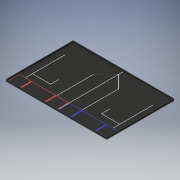
# Autodesk Inventor part: Field
Saved by Autodesk Inventor 2017 (Build 210142000, 142)
## iProperties
Created: 2017-04-14
Part Number: Field
Material: Generic
Document SubType Name: Modeling
Designer: Alex Tacescu
Density: 1 g/cm^3
Appearance: Rubber - Black
Author: Alex Tacescu
Autodesk Inventor part; units mm, degrees
ref_plane "YZ Plane" through (0, 0, 0) normal (1, 0, 0) x (0, 1, 0)
ref_plane "XZ Plane" through (0, 0, 0) normal (0, 1, 0) x (-1, 0, 0)
ref_plane "XY Plane" through (0, 0, 0) normal (0, 0, 1) x (1, 0, 0)
sketch "Sketch1" plane through (0, 0, 0) normal (0, 1, 0) x (-1, 0, 0)
  line L0 (0, -1706.88) -> (0, 1706.88) projected
  line L1 (-2560.32, 0) -> (2560.32, 0) projected
  line L2 (1828.8, 1219.2) -> (-1828.8, 1219.2)
  line L3 (-1828.8, 1219.2) -> (-1828.8, -1219.2)
  line L4 (-1828.8, -1219.2) -> (1828.8, -1219.2)
  line L5 (1828.8, -1219.2) -> (1828.8, 1219.2)
  line L6 (1828.8, 1219.2) -> (-1828.8, -1219.2) construction
  line L7 (-1828.8, 1219.2) -> (1828.8, -1219.2) construction
  point P0 (0, 0)
  dimension "d0" = 2438.4
  dimension "d1" = 3657.6
  constraints: 12 end point, 2 midpoint, 2 parallel, 1 horizontal, 1 perpendicular
  measures "d0" distance of L2.end L3.end
  measures "d1" distance of L3.end L4.end
extrude "Extrusion1" add sketch "Sketch1" along normal blind 6.35
sketch "Sketch2" plane through (0, 6.35, 0) normal (0, 1, 0) x (1, 0, 0)
  line L0 (-1828.8, -1219.2) -> (1828.8, -1219.2) projected
  line L1 (1828.8, -1219.2) -> (1828.8, 1219.2) projected
  line L2 (1828.8, 1219.2) -> (-1828.8, 1219.2) projected
  line L3 (-1828.8, 1219.2) -> (-1828.8, -1219.2) projected
  line L4 (-1816.1, 1206.5) -> (1816.1, 1206.5)
  line L5 (1816.1, 1206.5) -> (1816.1, -1206.5)
  line L6 (1816.1, -1206.5) -> (-1816.1, -1206.5)
  line L7 (-1816.1, -1206.5) -> (-1816.1, 1206.5)
  point P0 (0, 0)
  dimension "d4" = 12.7
  constraints: 8 end point, 3 other
  measures "d4" distance between parallel lines of L2 L4
extrude "Extrusion2" add sketch "Sketch2" along normal blind 63.5
sketch "Sketch4" plane through (0, 6.35, 0) normal (0, 1, 0) x (1, 0, 0)
  line L0 (1816.1, -1206.5) -> (1816.1, 1206.5) projected
  line L1 (1816.1, 1206.5) -> (-1816.1, 1206.5) projected
  line L2 (-1816.1, 1206.5) -> (-1816.1, -1206.5) projected
  line L3 (-1816.1, -1206.5) -> (1816.1, -1206.5) projected
  line L4 (-1828.8, -1219.2) -> (1828.8, -1219.2) projected
  line L5 (-1828.8, 1219.2) -> (-1828.8, -1219.2) projected
  line L6 (1828.8, 1219.2) -> (-1828.8, 1219.2) projected
  line L7 (1828.8, -1219.2) -> (1828.8, 1219.2) projected
  line L8 (-1816.1, -1206.5) -> (-1358.9, -1206.5)
  line L9 (-1358.9, -1206.5) -> (-1358.9, -749.3)
  line L10 (-1358.9, -749.3) -> (-1816.1, -749.3)
  line L11 (-1816.1, -749.3) -> (-1816.1, -1206.5)
  line L12 (-1790.7, -774.7) -> (-1384.3, -774.7)
  line L13 (-1384.3, -774.7) -> (-1384.3, -1181.1)
  line L14 (-1384.3, -1181.1) -> (-1790.7, -1181.1)
  line L15 (-1790.7, -1181.1) -> (-1790.7, -774.7)
  line L16 (0, 1706.88) -> (0, -1706.88) projected
  line L17 (2560.32, 0) -> (-2560.32, 0) projected
  line L18 (-1358.9, -1206.5) -> (-469.9, -1206.5)
  line L19 (-469.9, -1206.5) -> (-469.9, -749.3)
  line L20 (-469.9, -749.3) -> (-1358.9, -749.3)
  line L21 (-1358.9, -749.3) -> (-1358.9, -1206.5)
  line L22 (-469.9, -749.3) -> (-12.7, -749.3)
  line L23 (-12.7, -749.3) -> (-12.7, -1206.5)
  line L24 (-12.7, -1206.5) -> (-469.9, -1206.5)
  line L25 (-469.9, -1206.5) -> (-469.9, -749.3)
  line L26 (-495.3, -774.7) -> (-1333.5, -774.7)
  line L27 (-1333.5, -774.7) -> (-1333.5, -1181.1)
  line L28 (-1333.5, -1181.1) -> (-495.3, -1181.1)
  line L29 (-495.3, -1181.1) -> (-495.3, -774.7)
  line L30 (-444.5, -774.7) -> (-38.1, -774.7)
  line L31 (-38.1, -774.7) -> (-38.1, -1181.1)
  line L32 (-38.1, -1181.1) -> (-444.5, -1181.1)
  line L33 (-444.5, -1181.1) -> (-444.5, -774.7)
  line L34 (-12.7, -1206.5) -> (0, -1206.5)
  line L35 (0, -1206.5) -> (0, 609.6)
  line L36 (0, 609.6) -> (-12.7, 609.6)
  line L37 (-12.7, 609.6) -> (-12.7, -1206.5)
  line L38 (-1574.8, -749.3) -> (-1600.2, -749.3)
  point P0 (0, 0)
  dimension "d7" = 457.2
  dimension "d8" = 25.4
  dimension "d9" = 889
  dimension "d10" = 457.2
  dimension "d11" = 25.4
  dimension "d12" = 25.4
  dimension "d13" = 609.6
  constraints: 58 end point, 12 parallel, 8 perpendicular, 5 horizontal, 4 collinear, 3 point on line, 6 other
  measures "d7" distance of L8.end L9.end
  measures "d8" distance between parallel lines of L10 L12
  measures "d9" distance of L19.end L20.end
  measures "d10" distance of L19.end L22.end
  measures "d11" distance between parallel lines of L27 L9
  measures "d12" distance between parallel lines of L29 L25
  measures "d13" distance between parallel lines of L36 L6
extrude "Extrusion3" add sketch "Sketch4" along normal blind 0.254 contours L3 L19 L22 L23 | L3 L9 L20 L19 | L3 L2 L10 L9
sketch "Sketch7" plane through (0, 6.35, 0) normal (0, 1, 0) x (1, 0, 0)
  line L0 (0, 1706.88) -> (0, -1706.88) projected
  line L1 (2560.32, 0) -> (-2560.32, 0) projected
  line L2 (-1816.1, -749.3) -> (-12.7, -749.3) projected
  line L3 (-12.7, -749.3) -> (-12.7, -1206.5) projected
  line L4 (-12.7, -1206.5) -> (1816.1, -1206.5) projected
  line L5 (1816.1, -1206.5) -> (1816.1, 1206.5) projected
  line L6 (1816.1, 1206.5) -> (-1816.1, 1206.5) projected
  line L7 (-1816.1, 1206.5) -> (-1816.1, -749.3) projected
  line L8 (-469.9, 590.804) -> (-444.5, 590.804)
  line L9 (-444.5, 590.804) -> (-444.5, -749.046)
  line L10 (-444.5, -749.046) -> (-469.9, -749.046)
  line L11 (-469.9, -749.046) -> (-469.9, 590.804)
  line L12 (-469.9, 590.804) -> (-17.9605, 1042.7435)
  line L13 (-17.9605, 1042.7435) -> (0, 1024.783)
  line L14 (-444.5, -1181.1) -> (-444.5, -774.7) projected
  line L15 (0, 1024.783) -> (-444.5, 580.283)
  line L16 (-1600.2, -749.046) -> (-1574.8, -749.046)
  line L17 (-1574.8, -749.046) -> (-1574.8, 698.5)
  line L18 (-1574.8, 698.5) -> (-1600.2, 698.5)
  line L19 (-1600.2, 698.5) -> (-1600.2, -749.046)
  line L20 (-12.7, -749.3) -> (-1816.1, -749.3) projected
  line L21 (-1574.8, -520.7) -> (-914.4, -520.7)
  line L22 (-914.4, -520.7) -> (-914.4, -495.3)
  line L23 (-914.4, -495.3) -> (-1574.8, -495.3)
  line L24 (-1574.8, -495.3) -> (-1574.8, -520.7)
  line L25 (-914.4, -495.3) -> (-939.8, -495.3)
  line L26 (-939.8, -495.3) -> (-939.8, -209.55)
  line L27 (-939.8, -209.55) -> (-914.4, -209.55)
  line L28 (-914.4, -209.55) -> (-914.4, -495.3)
  point P0 (0, 0)
  dimension "d21" = 1339.85
  dimension "d22" = 25.4
  dimension "d23" = 0.254
  dimension "d24" = 135
  dimension "d25" = 508
  dimension "d26" = 0.254
  dimension "d27" = 215.9
  dimension "d28" = 228.6
  dimension "d29" = 285.75
  dimension "d31" = 635
  constraints: 38 end point, 9 parallel, 5 perpendicular, 4 equal length, 4 horizontal, 3 point on line, 1 collinear
  measures "d21" distance of L8.end L9.end
  measures "d22" distance of L9.end L10.end
  measures "d23" distance between parallel lines of L2 L10
  measures "d24" angle of L9 L15
  measures "d25" distance between parallel lines of L6 L18
  measures "d26" distance between parallel lines of L20 L16
  measures "d27" distance between parallel lines of L7 L19
  measures "d28" distance between parallel lines of L20 L21
  measures "d29" distance of L25.end L26.end
  measures "d31" distance between parallel lines of L17 L26
extrude "Extrusion5" add sketch "Sketch7" along normal blind 0.254 contours L15 L9 L8 L12 L13 | L9 L1 L11 L8 | L9 L10 L11 L1 | L19 L18 L17 L1 | L1 L17 L16 L19 | L23 L22 L21 L17 | L26 L27 L28 L23
mirror "Mirror1" about plane through (0, 0, 0) normal (1, 0, 0) of "Extrusion3", "Extrusion5"
sketch "Sketch5" plane through (0, 6.35, 0) normal (0, 1, 0) x (1, 0, 0)
  line L0 (-1384.3, -774.7) -> (-1384.3, -1181.1) projected
  line L1 (-1384.3, -1181.1) -> (-1790.7, -1181.1) projected
  line L2 (-1790.7, -1181.1) -> (-1790.7, -774.7) projected
  line L3 (-1790.7, -774.7) -> (-1384.3, -774.7) projected
  line L4 (-495.3, -774.7) -> (-495.3, -1181.1) projected
  line L5 (-495.3, -1181.1) -> (-1333.5, -1181.1) projected
  line L6 (-1333.5, -1181.1) -> (-1333.5, -774.7) projected
  line L7 (-1333.5, -774.7) -> (-495.3, -774.7) projected
  line L8 (-38.1, -774.7) -> (-38.1, -1181.1) projected
  line L9 (-38.1, -1181.1) -> (-444.5, -1181.1) projected
  line L10 (-444.5, -1181.1) -> (-444.5, -774.7) projected
  line L11 (-444.5, -774.7) -> (-38.1, -774.7) projected
  line L12 (-12.7, -1206.5) -> (-12.7, -749.3) projected
  line L13 (-12.7, -749.3) -> (-1816.1, -749.3) projected
  line L14 (-1816.1, -1206.5) -> (-1816.1, -749.3) projected
  line L15 (-12.7, -1206.5) -> (-1816.1, -1206.5) projected
  line L16 (1384.3, -774.7) -> (1384.3, -1181.1) projected
  line L17 (1790.7, -774.7) -> (1384.3, -774.7) projected
  line L18 (1790.7, -1181.1) -> (1790.7, -774.7) projected
  line L19 (1384.3, -1181.1) -> (1790.7, -1181.1) projected
  line L20 (495.3, -774.7) -> (495.3, -1181.1) projected
  line L21 (1333.5, -774.7) -> (495.3, -774.7) projected
  line L22 (1333.5, -1181.1) -> (1333.5, -774.7) projected
  line L23 (495.3, -1181.1) -> (1333.5, -1181.1) projected
  line L24 (38.1, -774.7) -> (38.1, -1181.1) projected
  line L25 (444.5, -774.7) -> (38.1, -774.7) projected
  line L26 (444.5, -1181.1) -> (444.5, -774.7) projected
  line L27 (38.1, -1181.1) -> (444.5, -1181.1) projected
  line L28 (12.7, -1206.5) -> (12.7, -749.3) projected
  line L29 (1816.1, -1206.5) -> (12.7, -1206.5) projected
  line L30 (1816.1, -749.3) -> (1816.1, -1206.5) projected
  line L31 (12.7, -749.3) -> (1816.1, -749.3) projected
  line L32 (12.7, -749.3) -> (1816.1, -749.3) projected
  line L33 (1816.1, -749.3) -> (1816.1, 1206.5) projected
  line L34 (1816.1, 1206.5) -> (-1816.1, 1206.5) projected
  line L35 (-1816.1, 1206.5) -> (-1816.1, -749.3) projected
  line L36 (-1816.1, -749.3) -> (-12.7, -749.3) projected
  line L37 (-12.7, -749.3) -> (-12.7, -1206.5) projected
  line L38 (-12.7, -1206.5) -> (12.7, -1206.5) projected
  line L39 (12.7, -1206.5) -> (12.7, -749.3) projected
  line L40 (-12.7, -1206.5) -> (12.7, -1206.5)
  line L41 (12.7, -1206.5) -> (12.7, 1206.5)
  line L42 (12.7, 1206.5) -> (-12.7, 1206.5)
  line L43 (-12.7, 1206.5) -> (-12.7, -1206.5)
  line L44 (-12.6746, -1206.4746) -> (12.6746, -1206.4746)
  line L45 (12.6746, -1206.4746) -> (12.6746, 1206.4746)
  line L46 (12.6746, 1206.4746) -> (-12.6746, 1206.4746)
  line L47 (-12.6746, 1206.4746) -> (-12.6746, -1206.4746)
  point P0 (0, 0)
  dimension "d18" = 0.0254
  constraints: 16 end point, 4 parallel, 2 perpendicular, 1 collinear, 1 horizontal, 1 point on line, 3 other
  measures "d18" distance between parallel lines of L43 L47
extrude "Extrusion4" add sketch "Sketch5" along normal blind 0.254 contours L47 L46 L45 L44
equation "\"d11\" = d8"
equation "\"d12\" = d11"
body "Solid1"
